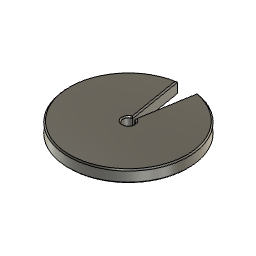
Pendulum String Clip v3 (Autodesk Fusion 360 design; units mm, degrees)
Autodesk Fusion 360 part; units mm, degrees
sketch "Sketch1" plane through (0, 0, 0) normal (0, 0, 1) x (1, 0, 0) in component "String Clip"
  circle A0 centre (0, 0) radius 5
  circle A1 centre (0, 0) radius 0.45
  line L0 (0, 0) -> (5, 0) construction
  line L1 (0, 0) -> (5, 0) construction
  line L2 (0, 0) -> (0, 0.45)
  line L3 (0, 0) -> (-0.8333, 4.9301)
  line L4 (0, 0) -> (5, 0) construction
  line L5 (0, 0) -> (0.8333, 4.9301)
  line L6 (0, 0) -> (5, 0) construction
  dimension "d1" = 10
  dimension "d2" = 0.9
  dimension "d11" = 99.594
  dimension "d12" = 80.406
  dimension "d13" = 5
  dimension "d16" = 5
  constraint coincident A0.centre A1.centre
  constraint concentric A0 A1
  constraint horizontal L0
  constraint horizontal L1
  constraint coincident A1 L2.end
  constraint perpendicular L1 L2
  constraint horizontal L4
  constraint horizontal L6
  measures "d1" diameter of A0
  measures "d2" diameter of A1
  measures "d11" angle of L3 L4
  measures "d12" angle of L5 L6
  measures "d13" distance of A0.centre L5.end
  measures "d16" distance of A0.centre L3.end
extrude "Extrude1" add sketch "Sketch1" along normal blind 1 contours A0 A1 L3 L5 picked at (-2.1775, 2.7069) in component "String Clip"
chamfer "Chamfer1" distance 0.1 angle 45 2 faces at (-2.1775, 2.7069, 1) (-2.1775, 2.7069, 0) in component "String Clip"
component "String Clip" placed x (1, 0, 0) y (0, 1, 0) z (0, 0, 1) at (0, 0, 0)
equation "d1 = DiskDiameter"
equation "d2 = StringDiameter"
equation "d6 = DiskHeight"
equation "DiskDiameter = 10 mm"
equation "StringDiameter = 0.9 mm"
equation "GapWidth = 0.15 mm"
equation "d11 = 90 deg + GapAngle / 2"
equation "d12 = 90 deg - GapAngle / 2"
equation "d13 = DiskDiameter / 2"
equation "GapAngle = asin(GapWidth / StringDiameter) * 2"
equation "d16 = DiskDiameter / 2"
equation "DiskHeight = 1 mm"
named bodies: "Clip"
